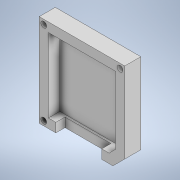
# Autodesk Inventor part: SpeakerHolder
Saved by Autodesk Inventor 2020 (Build 240168000, 168)
## iProperties
Created: 2019-05-29
Part Number: SpeakerHolder
Material: Generic
Document SubType Name: Modeling
Designer: Dammy
Density: 1 g/cm^3
Appearance: Default
Author: Dammy
Autodesk Inventor part; units mm, degrees
ref_plane "YZ Plane" through (0, 0, 0) normal (1, 0, 0) x (0, 1, 0)
ref_plane "XZ Plane" through (0, 0, 0) normal (0, 1, 0) x (-1, 0, 0)
ref_plane "XY Plane" through (0, 0, 0) normal (0, 0, 1) x (1, 0, 0)
sketch "Sketch1" plane through (0, 0, 0) normal (0, 0, 1) x (1, 0, 0)
  line L0 (11.825, -16.125) -> (-11.825, -16.125)
  line L1 (-14.625, -13.325) -> (-14.625, 16.125)
  line L2 (-14.625, 16.125) -> (14.625, 16.125)
  line L3 (14.625, 16.125) -> (14.625, -13.325)
  line L4 (14.625, -16.125) -> (-14.625, 16.125) construction
  line L5 (-14.625, -16.125) -> (14.625, 16.125) construction
  line L6 (11.825, -16.125) -> (14.625, -13.325)
  line L7 (-14.625, -13.325) -> (-14.625, -16.125)
  line L8 (-14.625, -16.125) -> (-11.825, -16.125)
  point P0 (0, 0)
  dimension "d0" = 29.25
  dimension "d1" = 32.25
  dimension "d24" = 2.8
  dimension "d25" = 2.8
  constraints: 18 end point, 4 point on line, 2 midpoint, 2 parallel, 2 perpendicular, 1 horizontal, 1 vertical
  measures "d0" distance of L1.end L2.end
  measures "d1" distance of L5.start L1.end
  measures "d24" distance of L0.start L4.start
  measures "d25" distance of L3.end L4.start
extrude "Extrusion1" add sketch "Sketch1" along normal blind 5
shell "Shell2" thickness 4 outward yes removed faces 1 at (-4.875, -3.5083, 5)
sketch "Sketch3" plane through (0, 0, 5) normal (0, 0, 1) x (1, 0, 0)
  line L0 (18.625, 20.125) -> (-18.625, 20.125) construction
  line L1 (-14.625, 16.125) -> (14.625, 16.125) construction
  line L2 (-18.625, 20.125) -> (-14.625, 16.125) construction
  line L3 (18.625, -14.9819) -> (18.625, 20.125) construction
  line L4 (14.625, 16.125) -> (18.625, 20.125) construction
  line L5 (11.825, -16.125) -> (-14.625, -16.125) construction
  circle A0 centre (-16.625, 18.125) radius 1.25
  circle A1 centre (16.625, 18.125) radius 1.25
  line L6 (-14.625, -16.125) -> (11.825, -16.125) construction
  line L7 (-18.625, 20.125) -> (-18.625, -20.125) construction
  line L8 (-14.625, -16.125) -> (-18.625, -20.125) construction
  circle A2 centre (-16.625, -18.125) radius 1.25
  point P0 (0, 0)
  point P1 (-11.825, -16.125)
  dimension "d14" = 2.5
  dimension "d15" = 2.5
  dimension "d26" = 2.5
  constraints: 6 end point, 3 centre point, 3 midpoint
  measures "d14" diameter of A0
  measures "d15" diameter of A1
  measures "d26" diameter of A2
extrude "Extrusion3" cut sketch "Sketch3" against normal through all
sketch "Sketch4" plane through (0, 0, 5) normal (0, 0, 1) x (1, 0, 0)
  line L0 (-18.625, -20.125) -> (13.4819, -20.125) projected
  line L1 (11.825, -16.125) -> (-14.625, -16.125) projected
  line L2 (8.625, -20.125) -> (-11.375, -20.125)
  line L3 (-11.375, -20.125) -> (-11.375, -16.125)
  line L4 (-11.375, -16.125) -> (8.625, -16.125)
  line L5 (8.625, -16.125) -> (8.625, -20.125)
  line L6 (-18.625, 20.125) -> (-18.625, -20.125) projected
  point P0 (0, 0)
  point P1 (-13.4819, -20.125)
  point P2 (14.625, -16.125)
  point P3 (-11.825, -16.125)
  point P4 (8.625, -16.125)
  dimension "d19" = 20
  dimension "d20" = 4
  dimension "d29" = 7.25
  constraints: 8 end point, 2 parallel, 2 point on line, 1 horizontal, 1 perpendicular
  measures "d19" distance of L3.end L4.end
  measures "d20" distance between parallel lines of L0 L1
  measures "d29" distance between parallel lines of L6 L3
extrude "Extrusion4" cut sketch "Sketch4" against normal blind 4
sketch "Sketch5" plane through (0, 0, -4) normal (0, 0, -1) x (-1, 0, 0)
  line L0 (-18.625, 20.125) -> (18.625, 20.125) projected
  line L1 (18.625, -20.125) -> (-13.4819, -20.125) projected
  line L2 (-18.625, 20.125) -> (18.625, 20.125)
  line L3 (18.625, 20.125) -> (18.625, -20.125)
  line L4 (18.625, -20.125) -> (-18.625, -20.125)
  line L5 (-18.625, -20.125) -> (-18.625, 20.125)
  point P0 (0, 0)
  constraints: 8 end point, 2 parallel, 1 horizontal, 1 perpendicular
extrude "Extrusion5" cut sketch "Sketch5" against normal blind 2
equation "\"d25\" = d24"
equation "\"d26\" = d14"
body "Solid1"
